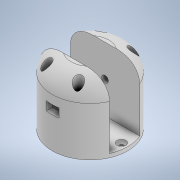
# Autodesk Inventor part: tilt_1_base
Saved by Autodesk Inventor 2022.3 (Build 263350000, 350)
## iProperties
Created: 2022-05-28
Part Number: tilt_1_base
Material: Generic
Document SubType Name: Modeling
Designer: Mlees
Density: 1 g/cm^3
Appearance: Default
Author: Mlees
Autodesk Inventor part; units mm, degrees
ref_plane "YZ Plane" through (0, 0, 0) normal (1, 0, 0) x (0, 1, 0)
ref_plane "XZ Plane" through (0, 0, 0) normal (0, 1, 0) x (-1, 0, 0)
ref_plane "XY Plane" through (0, 0, 0) normal (0, 0, 1) x (1, 0, 0)
sketch "Sketch1" plane through (0, 0, 0) normal (0, 1, 0) x (-1, 0, 0)
  circle A0 centre (0, 0) radius 30
  circle A1 centre (-25, 0) radius 1.5
  circle A2 centre (-12.5, -21.6506) radius 1.5
  circle A3 centre (12.5, -21.6506) radius 1.5
  circle A4 centre (25, 0) radius 1.5
  circle A5 centre (12.5, 21.6506) radius 1.5
  circle A6 centre (-12.5, 21.6506) radius 1.5
  dimension "d0" = 60
  dimension "d2" = 3
  dimension "d5" = 360
  constraints: 7 centre point, 1 coincident, 13 other
  measures "d0" diameter of A0
  measures "d2" diameter of A1
extrude "Extrusion1" add sketch "Sketch1" along normal blind 3
fillet "Fillet1" radius 2 6 edges at (-11, 3, 21.6506) (-23.5, 3, 0) (-11, 3, -21.6506) (14, 3, -21.6506) (26.5, 3, 0) (14, 3, 21.6506) inverted yes
sketch "Sketch5" plane through (0, 3, 0) normal (0, 1, 0) x (1, 0, 0)
  circle A0 centre (0, 0) radius 30
  constraints: 1 centre point, 1 coincident
extrude "Extrusion5" add sketch "Sketch5" along normal blind 50.8
fillet "Fillet3" radius 15 1 edges at (-30, 53.8, 0)
sketch "Sketch6" plane through (0, 53.8, 0) normal (0, 1, 0) x (1, 0, 0)
  circle A0 centre (-25, 0) radius 1.5 projected
  circle A1 centre (-25, 0) radius 3.5
  circle A2 centre (0, 0) radius 15
  circle A3 centre (-12.5, -21.6506) radius 3.5
  circle A4 centre (12.5, -21.6506) radius 3.5
  circle A5 centre (25, 0) radius 3.5
  circle A6 centre (12.5, 21.6506) radius 3.5
  circle A7 centre (-12.5, 21.6506) radius 3.5
  dimension "d29" = 360
  constraints: 7 centre point, 2 coincident, 13 other
extrude "Extrusion6" cut sketch "Sketch6" against normal blind 50.8 contours A0 | A1 | A3 | A4 | A5 | A6 | A7
sketch "Sketch9" plane through (0, 53.8, 0) normal (0, 1, 0) x (1, 0, 0)
  line L0 (0, 12) -> (-27.4955, 12)
  circle A0 centre (0, 0) radius 30 projected
  line L1 (0, 12) -> (27.4955, 12)
  line L2 (0, -12) -> (27.4955, -12)
  line L3 (0, -12) -> (-27.4955, -12)
  arc A1 (-27.4955, 12) -> (-27.4955, -12) centre (0, 0) ccw
  arc A2 (27.4955, -12) -> (27.4955, 12) centre (0, 0) ccw
  dimension "d41" = 12
  dimension "d42" = 12
  constraints: 8 end point, 8 point on circle, 2 centre point, 2 concentric, 2 point on line
  measures "d41" distance of point (0, 0) L0.start
  measures "d42" distance of A0.centre L2.start
extrude "Extrusion9" cut sketch "Sketch9" against normal blind 50.8 contours L1 A0 L2 L3 L0
ref_plane "Work Plane2" through (-9, 53.8, 0) normal (0, 0, 1) x (1, 0, 0)
sketch "Sketch10" plane through (-9, 53.8, -12) normal (0, 0, 1) x (1, 0, 0)
  line L0 (0, 0) -> (18, 0) projected
  line L1 (-18.4955, -50.8) -> (36.4955, -50.8) projected
  circle A0 centre (9, -25.4) radius 2.625
  point P0 (9, -53.8)
  dimension "d45" = 5.25
  constraints: 1 centre point
  measures "d45" diameter of A0
extrude "Extrusion10" cut sketch "Sketch10" along normal mid plane 100
ref_plane "Work Plane3" through (0, 0, 30) normal (0, 0, 1) x (1, 0, 0)
sketch "Sketch11" plane through (0, 0, 30) normal (0, 0, 1) x (1, 0, 0)
  circle A0 centre (0, 28.4) radius 2.625 projected
  line L0 (0, 31.9) -> (5, 31.9)
  line L1 (0, 24.9) -> (-5, 24.9)
  line L2 (-5, 24.9) -> (5, 24.9)
  line L3 (5, 24.9) -> (5, 31.9)
  line L4 (5, 31.9) -> (-5, 31.9)
  line L5 (-5, 31.9) -> (-5, 24.9)
  point P0 (0, 0)
  dimension "d49" = 5
  dimension "d51" = 5
  constraints: 12 end point, 2 parallel, 1 horizontal, 1 perpendicular
  measures "d49" distance of L0.start L0.end
  measures "d51" distance of L1.start L1.end
extrude "Extrusion11" cut sketch "Sketch11" against normal blind 5
ref_plane "Work Plane4" through (0, 0, -30) normal (0, 0, -1) x (-1, 0, 0)
sketch "Sketch12" plane through (0, 0, -30) normal (0, 0, -1) x (-1, 0, 0)
  circle A0 centre (0, 28.4) radius 2.625 projected
  line L0 (5, 31.9) -> (-5, 31.9) projected
  line L1 (-5, 31.9) -> (-5, 24.9) projected
  line L2 (0, 31.9) -> (-5, 31.9)
  line L3 (-5, 24.9) -> (5, 24.9) projected
  line L4 (-5, 31.9) -> (-5, 24.9)
  line L5 (-5, 24.9) -> (5, 24.9)
  line L6 (5, 24.9) -> (5, 31.9) projected
  line L7 (5, 24.9) -> (5, 31.9)
  line L8 (5, 31.9) -> (0, 31.9)
  point P0 (0, 0)
  constraints: 10 end point, 4 perpendicular, 1 collinear, 1 midpoint
extrude "Extrusion12" cut sketch "Sketch12" against normal blind 5
body "Solid1"
